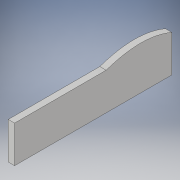
# Autodesk Inventor part: Inboard Wing Brace
Saved by Autodesk Inventor 2018 (Build 220112000, 112)
## iProperties
Created: 2018-08-13
Part Number: Inboard Wing Brace
Material: Generic
Document SubType Name: Modeling
Designer: Michael Gunderman
Density: 1 g/cm^3
Appearance: Default
Author: Michael Gunderman
Autodesk Inventor part; units mm, degrees
ref_plane "YZ Plane" through (0, 0, 0) normal (1, 0, 0) x (0, 1, 0)
ref_plane "XZ Plane" through (0, 0, 0) normal (0, 1, 0) x (-1, 0, 0)
ref_plane "XY Plane" through (0, 0, 0) normal (0, 0, 1) x (1, 0, 0)
sketch "Sketch1" plane through (0, 0, 0) normal (1, 0, 0) x (0, 1, 0)
  line L0 (0, 0) -> (35, 0)
  line L1 (35, 0) -> (35, -86.8367)
  line L2 (35, -149) -> (0, -149)
  line L3 (0, -149) -> (0, 0)
  spline S0 degree 2 poles (35, -149) (46.832, -120.836) (35, -86.8367) knots 0 0 0 1 1 1
  point P0 (0, -76.4686)
  point P1 (40.9046, -120.7367)
  dimension "d0" = 35
  dimension "d1" = 149
  constraints: 8 end point, 2 horizontal, 1 perpendicular, 1 point on line, 1 vertical, 4 other
  measures "d0" distance of L0.start L0.end
  measures "d1" distance of L0.end L2.start
extrude "Extrusion1" add sketch "Sketch1" against normal blind 6
body "Solid1"
